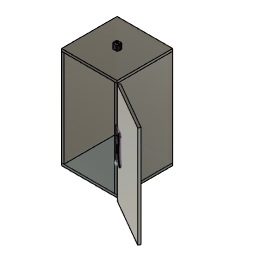
Mixer v4 (Autodesk Fusion 360 design; units mm, degrees)
Autodesk Fusion 360 part; units mm, degrees
sketch "Sketch1" plane through (0, 0, 0) normal (0, 1, 0) x (1, 0, 0)
  line L0 (0, 0) -> (0, -5)
  line L1 (0, -5) -> (115, -5)
  line L2 (115, -5) -> (115, 0)
  line L3 (115, 0) -> (0, 0)
  constraint coincident L0.start L3.end
  constraint vertical L0
  constraint perpendicular L0 L1
  constraint perpendicular L1 L2
  constraint perpendicular L0 L3
extrude "Extrude1" add sketch "Sketch1" along normal blind 115 makes body 1
sketch "Sketch6" plane through (0, 0, 5) normal (0, 0, 1) x (-1, 0, 0)
  line L0 (0, 0) -> (-115, 0)
  line L1 (-115, 0) -> (-115, -115)
  line L2 (-115, -115) -> (0, -115)
  line L3 (0, -115) -> (0, 0)
  line L4 (0, -115) -> (-5, -115)
  line L5 (-5, -115) -> (-5, 0)
  line L6 (-5, 0) -> (0, 0)
  line L7 (0, 0) -> (0, -115)
  constraint horizontal L4
  constraint vertical L5
  constraint horizontal L6
  constraint vertical L7
  constraint coincident L0 L5.end
  constraint coincident L2.end L3.start
extrude "Extrude2" add sketch "Sketch6" along normal blind 200 separate body contours L0 L2 L3 L4 L5 L6 L7 makes body 2
sketch "Sketch7" plane through (0, 0, 5) normal (0, 0, 1) x (-1, 0, 0)
  line L0 (0, 0) -> (-115, 0)
  line L1 (-115, 0) -> (-115, -115)
  line L2 (-115, -115) -> (0, -115)
  line L3 (0, -115) -> (0, 0)
  line L4 (-115, -115) -> (-110, -115)
  line L5 (-110, -115) -> (-110, 0)
  line L6 (-110, 0) -> (-115, 0)
  line L7 (-115, 0) -> (-115, -115)
  constraint horizontal L4
  constraint vertical L5
  constraint horizontal L6
  constraint vertical L7
  constraint coincident L0 L5.end
  constraint coincident L1.end L2.start
extrude "Extrude3" add sketch "Sketch7" along normal blind 200 separate body contours L0 L1 L2 L4 L5 L6 L7 makes body 3
sketch "bottom" plane through (0, 0, 5) normal (0, 0, 1) x (-1, 0, 0)
  line L0 (0, 0) -> (-115, 0)
  line L1 (-115, 0) -> (-115, -115)
  line L2 (-115, -115) -> (0, -115)
  line L3 (0, -115) -> (0, 0)
sketch "b_wall" plane through (0, 0, 5) normal (0, 0, 1) x (1, 0, 0)
  line L0 (5, 115) -> (110, 115)
  line L1 (110, 115) -> (110, 110)
  line L2 (110, 110) -> (5, 110)
  line L3 (5, 110) -> (5, 115)
  constraint horizontal L0
  constraint vertical L1
  constraint horizontal L2
  constraint vertical L3
extrude "Extrude4" add sketch "b_wall" along normal blind 200 separate body makes body 4
sketch "Sketch11" plane through (0, 0, 205) normal (0, 0, 1) x (-1, 0, 0)
  line L0 (0, 0) -> (-5, 0)
  line L1 (-5, 0) -> (-5, -115)
  line L2 (-5, -115) -> (0, -115)
  line L3 (0, -115) -> (0, 0)
  line L4 (0, -115) -> (-115, -115)
  line L5 (-115, -115) -> (-115, 0)
  line L6 (-115, 0) -> (0, 0)
  line L7 (0, 0) -> (0, -115)
  constraint horizontal L4
  constraint vertical L5
  constraint horizontal L6
  constraint vertical L7
  constraint coincident L2.end L3.start
sketch "top" plane through (0, 0, 0) normal (0, 1, 0) x (-1, 0, 0)
  line L0 (-115, 205) -> (0, 205)
  line L1 (0, 205) -> (0, 210)
  line L2 (0, 210) -> (-115, 210)
  line L3 (-115, 210) -> (-115, 205)
  constraint horizontal L0
  constraint vertical L1
  constraint horizontal L2
  constraint vertical L3
extrude "Extrude6" add sketch "top" along normal blind 115 separate body makes body 5
sketch "Sketch16" plane through (0, 0, 210) normal (0, 0, 1) x (-1, 0, 0)
  line L0 (0, 0) -> (-115, 0)
  line L1 (-115, 0) -> (-115, -115)
  line L2 (-115, -115) -> (0, -115)
  line L3 (0, -115) -> (0, 0)
  line L4 (-51.5, -62.5) -> (-63.5, -62.5)
  line L5 (-63.5, -62.5) -> (-63.5, -52.5)
  line L6 (-63.5, -52.5) -> (-51.5, -52.5)
  line L7 (-51.5, -52.5) -> (-51.5, -62.5)
  circle A0 centre (-57.5, -57.5) radius 6
  constraint horizontal L4
  constraint vertical L5
  constraint horizontal L6
  constraint vertical L7
  constraint tangent L7 A0
form "Form1" [no effect]
emboss "Emboss1" depth -10 profiles "Sketch16" section 1 contours L4 L6 A0 onto face at (38.3333, 76.6667, 210) on bodies 5 bodies 5
copy_body "Body->Comp1" bodies 3 removing the originals makes body 6 in component "Component"
copy_body "Body->Comp2" bodies 5 removing the originals makes body 7 in component "Component'"
copy_body "Body->Comp3" bodies 2 removing the originals makes body 8 in component "Component''"
copy_body "Body->Comp4" bodies 1 removing the originals makes body 9 in component "Component'''"
copy_body "Body->Comp5" bodies 4 removing the originals makes body 10 in component "Component''''"
sketch "Sketch17" plane through (0, 110, 0) normal (0, -1, 0) x (1, 0, 0)
  line L0 (5, 5) -> (110, 5)
  line L1 (110, 5) -> (110, 205)
  line L2 (110, 205) -> (5, 205)
  line L3 (5, 205) -> (5, 5)
sketch "Sketch18" plane through (57.5, 110, 105) normal (0, -1, 0) x (1, 0, 0)
  circle A0 centre (-40, -90) radius 5
hole "Hole1" at (17.5, 110, 15) direction (0, 1, 0) diameter 6 depth 25 tip angle 118 bodies 10 in component "Component''''"
sketch "Sketch19" plane through (0, 0, 210) normal (0, 0, 1) x (-1, 0, 0)
  arc A0 (-54.1834, -62.5) -> (-54.1834, -52.5) centre (-57.5, -57.5) ccw
  line L0 (-54.1834, -62.5) -> (-60.8166, -62.5)
  arc A1 (-60.8166, -52.5) -> (-60.8166, -62.5) centre (-57.5, -57.5) ccw
  line L1 (-60.8166, -52.5) -> (-54.1834, -52.5)
  line L2 (0, 0) -> (-115, 0)
  line L3 (-115, 0) -> (-115, -115)
  line L4 (-115, -115) -> (0, -115)
  line L5 (0, -115) -> (0, 0)
  line L6 (0, 0) -> (-115, 0)
  line L7 (-115, 0) -> (-115, 5)
  line L8 (-115, 5) -> (0, 5)
  line L9 (0, 5) -> (0, 0)
  constraint horizontal L6
  constraint vertical L7
  constraint horizontal L8
  constraint vertical L9
  constraint coincident L2.start L5.end
extrude "Extrude1'" add sketch "Sketch19" against normal blind 210 separate body contours L2 L6 L7 L8 L9 makes body 11 in component "Component'''''"
mesh "Mesh1" [no effect]
mesh "Mesh2" [no effect]
mesh "Mesh3" [no effect]
copy_body "Body->Comp1'" bodies 6 removing the originals makes body 12 in component "Component''''''"
sketch "Sketch20" plane through (0, 0, 5) normal (0, 0, 1) x (-1, 0, 0)
  circle A0 centre (-57.5852, -57.6371) radius 1.9308
sketch "Sketch21" plane through (0, 110, 0) normal (0, -1, 0) x (1, 0, 0)
mesh "Mesh4" [no effect]
hole "Hole1'" at (115, 13.2931, 125.8948) direction (-1, 0, 0) diameter 2.529 depth 5 tip angle 118 bodies 12 in component "Component''''''"
thread "Thread1" "ISO Metric profile 3.0 M3x0.5 6H" in component "Component''''''"
hole "Hole2" at (115, 12.1237, 110.3038) direction (-1, 0, 0) diameter 2.529 depth 5 tip angle 118 bodies 12 in component "Component''''''"
thread "Thread2" "ISO Metric profile 3.0 M3x0.5 6H" in component "Component''''''"
hole "Hole3" at (115, 13.2917, 94.6807) direction (-1, 0, 0) diameter 2.529 depth 5 tip angle 118 bodies 12 in component "Component''''''"
thread "Thread3" "ISO Metric profile 3.0 M3x0.5 6H" in component "Component''''''"
hole "Hole4" at (115, 12.1098, 79.0442) direction (-1, 0, 0) diameter 2.529 depth 5 tip angle 118 bodies 12 in component "Component''''''"
thread "Thread4" "ISO Metric profile 3.0 M3x0.5 6H" in component "Component''''''"
hole "Hole1''" at (105.2587, 0, 126.1707) direction (0, -1, 0) diameter 2.529 depth 5 tip angle 118 bodies 11 in component "Component'''''"
thread "Thread1'" "ISO Metric profile 3.0 M3x0.5 6H" in component "Component'''''"
hole "Hole2'" at (104.1553, 0, 110.1046) direction (0, -1, 0) diameter 2.529 depth 5 tip angle 118 bodies 11 in component "Component'''''"
thread "Thread2'" "ISO Metric profile 3.0 M3x0.5 6H" in component "Component'''''"
hole "Hole3'" at (105.3318, 0, 94.527) direction (0, -1, 0) diameter 2.529 depth 5 tip angle 118 bodies 11 in component "Component'''''"
thread "Thread3'" "ISO Metric profile 3.0 M3x0.5 6H" in component "Component'''''"
hole "Hole4'" at (104.1978, 0, 78.9126) direction (0, -1, 0) diameter 2.529 depth 5 tip angle 118 bodies 11 in component "Component'''''"
thread "Thread4'" "ISO Metric profile 3.0 M3x0.5 6H" in component "Component'''''"
mesh "Mesh5" [no effect]
component "Component" placed x (1, 0, 0) y (0, 1, 0) z (0, 0, 1) at (0, 0, 0)
component "Component'" placed x (1, 0, 0) y (0, 1, 0) z (0, 0, 1) at (0, 0, 0)
component "Component''" placed x (1, 0, 0) y (0, 1, 0) z (0, 0, 1) at (0, 0, 0)
component "Component'''" placed x (1, 0, 0) y (0, 1, 0) z (0, 0, 1) at (0, 0, 0)
component "Component''''" placed x (1, 0, 0) y (0, 1, 0) z (0, 0, 1) at (0, 0, 0)
component "Component'''''" placed x (-0.866025, 0.5, 0) y (-0.5, -0.866025, 0) z (0, 0, 1) at (221.453, -63.7531, 0.1084)
component "Component''''''" placed x (1, 0, 0) y (0, 1, 0) z (0, 0, 1) at (0, 0, 0) in component "Component"
